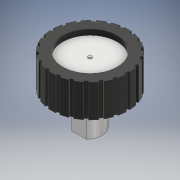
# Autodesk Inventor part: learnbotRueda
Saved by Autodesk Inventor 2017 (Build 210142000, 142)
## iProperties
Part Number: learnbotRueda
Material: Genérico
Document SubType Name: Modeling
Designer: rober
Density: 1 g/cm^3
Appearance: Valor por defecto
Author: rober
Autodesk Inventor part; units mm, degrees
ref_plane "YZ Plane" through (0, 0, 0) normal (1, 0, 0) x (0, 1, 0)
ref_plane "XZ Plane" through (0, 0, 0) normal (0, 1, 0) x (-1, 0, 0)
ref_plane "XY Plane" through (0, 0, 0) normal (0, 0, 1) x (1, 0, 0)
sketch "Boceto1" plane through (0, 0, 0) normal (0, 0, 1) x (1, 0, 0)
  circle A0 centre (0, 0.0001) radius 1.5
  line L0 (-0.1991, -2.0905) -> (0.1991, -2.0905)
  line L1 (0.3964, -2.0622) -> (0.7785, -1.9503)
  line L2 (0.9583, -1.8685) -> (1.2966, -1.6518)
  line L3 (0.7785, -1.9503) -> (0.7414, -1.8574)
  line L4 (0.9583, -1.8685) -> (0.9127, -1.7795)
  arc A1 (1.2349, -1.5731) -> (1.3772, -1.4502) centre (0, 0.0001) ccw
  arc A2 (-1.3773, -1.4502) -> (-1.235, -1.5731) centre (0, 0.0001) ccw
  arc A3 (-0.9128, -1.7795) -> (-0.7415, -1.8574) centre (0, 0.0001) ccw
  arc A4 (-0.3776, -1.964) -> (-0.1897, -1.9909) centre (0, 0.0001) ccw
  arc A5 (0.1896, -1.9909) -> (0.3775, -1.964) centre (0, 0.0001) ccw
  arc A6 (0.7414, -1.8574) -> (0.9127, -1.7795) centre (0, 0.0001) ccw
  line L5 (-1.2967, -1.6518) -> (-0.9584, -1.8685)
  line L6 (-0.7786, -1.9503) -> (-0.3964, -2.0622)
  line L7 (0.3775, -1.964) -> (0.3964, -2.0622)
  line L8 (0.1896, -1.9909) -> (0.1991, -2.0905)
  line L9 (-0.1897, -1.9909) -> (-0.1991, -2.0905)
  line L10 (-0.3776, -1.964) -> (-0.3964, -2.0622)
  line L11 (-1.235, -1.5731) -> (-1.2967, -1.6518)
  line L12 (-0.9584, -1.8685) -> (-0.9128, -1.7795)
  line L13 (-0.7415, -1.8574) -> (-0.7786, -1.9503)
  line L14 (1.2966, -1.6518) -> (1.2349, -1.5731)
  line L15 (-0.1991, 2.0906) -> (0.1991, 2.0906)
  line L16 (0.3964, 2.0623) -> (0.7785, 1.9504)
  line L17 (0.9583, 1.8686) -> (1.2966, 1.6519)
  line L18 (0.7785, 1.9504) -> (0.7414, 1.8575)
  line L19 (0.9583, 1.8686) -> (0.9127, 1.7796)
  arc A7 (1.3878, 1.4401) -> (1.2349, 1.5732) centre (-0.0001, 0) ccw
  arc A8 (-1.235, 1.5732) -> (-1.3879, 1.4401) centre (0, 0) ccw
  arc A9 (-0.7415, 1.8575) -> (-0.9128, 1.7796) centre (0, 0.0001) ccw
  arc A10 (-0.1897, 1.991) -> (-0.3776, 1.9641) centre (0, 0.0001) ccw
  arc A11 (0.3775, 1.9641) -> (0.1896, 1.991) centre (0, 0.0001) ccw
  arc A12 (0.9127, 1.7796) -> (0.7414, 1.8575) centre (0, 0.0001) ccw
  line L20 (-1.2967, 1.6519) -> (-0.9584, 1.8686)
  line L21 (-0.7786, 1.9504) -> (-0.3964, 2.0623)
  line L22 (0.3775, 1.9641) -> (0.3964, 2.0623)
  line L23 (0.1896, 1.991) -> (0.1991, 2.0906)
  line L24 (-0.1897, 1.991) -> (-0.1991, 2.0906)
  line L25 (-0.3776, 1.9641) -> (-0.3964, 2.0623)
  line L26 (-1.235, 1.5732) -> (-1.2967, 1.6519)
  line L27 (-0.9584, 1.8686) -> (-0.9128, 1.7796)
  line L28 (-0.7415, 1.8575) -> (-0.7786, 1.9504)
  line L29 (1.2966, 1.6519) -> (1.2349, 1.5732)
  line L30 (1.4461, -1.5227) -> (1.7075, -1.2223)
  line L31 (1.8148, -1.0565) -> (1.9828, -0.6915)
  line L32 (1.7075, -1.2223) -> (1.6262, -1.1641)
  line L33 (1.8148, -1.0565) -> (1.7284, -1.0062)
  arc A13 (1.6262, -1.1641) -> (1.7284, -1.0062) centre (0, 0.0001) ccw
  line L34 (1.3772, -1.4502) -> (1.4461, -1.5227)
  line L35 (2.039, -0.5021) -> (2.0973, -0.1046)
  line L36 (1.9828, -0.6915) -> (1.8884, -0.6585)
  line L37 (2.039, -0.5021) -> (1.9419, -0.4782)
  arc A14 (1.9975, -0.0996) -> (1.998, 0.0885) centre (0, 0.0001) ccw
  arc A15 (1.8884, -0.6585) -> (1.9419, -0.4782) centre (0, 0.0001) ccw
  line L38 (2.0973, -0.1046) -> (1.9975, -0.0996)
  line L39 (2.0979, 0.0929) -> (2.0427, 0.4873)
  line L40 (1.9878, 0.677) -> (1.8225, 1.0433)
  line L41 (2.0427, 0.4873) -> (1.9454, 0.4641)
  line L42 (1.9878, 0.677) -> (1.8932, 0.6448)
  arc A16 (1.9454, 0.4641) -> (1.8932, 0.6448) centre (0, 0.0001) ccw
  line L43 (1.998, 0.0885) -> (2.0979, 0.0929)
  arc A17 (1.7357, 0.9936) -> (1.6347, 1.1523) centre (0, 0.0001) ccw
  line L44 (1.8225, 1.0433) -> (1.7357, 0.9936)
  line L45 (1.7164, 1.2099) -> (1.4572, 1.5121)
  line L46 (1.4572, 1.5121) -> (1.3878, 1.4401)
  line L47 (1.6347, 1.1523) -> (1.7164, 1.2099)
  arc A18 (-1.3773, -1.4502) -> (-1.235, -1.5731) centre (0, 0.0001) ccw
  line L48 (-1.4462, -1.5227) -> (-1.7076, -1.2223)
  line L49 (-1.8149, -1.0565) -> (-1.9829, -0.6915)
  line L50 (-1.7076, -1.2223) -> (-1.6263, -1.1641)
  line L51 (-1.8149, -1.0565) -> (-1.7285, -1.0062)
  arc A19 (-1.7285, -1.0062) -> (-1.6263, -1.1641) centre (0, 0.0001) ccw
  line L52 (-1.3773, -1.4502) -> (-1.4462, -1.5227)
  line L53 (-2.0391, -0.5021) -> (-2.0974, -0.1046)
  line L54 (-1.9829, -0.6915) -> (-1.8885, -0.6585)
  line L55 (-2.0391, -0.5021) -> (-1.942, -0.4782)
  arc A20 (-1.9981, 0.0885) -> (-1.9976, -0.0996) centre (0, 0.0001) ccw
  arc A21 (-1.942, -0.4782) -> (-1.8885, -0.6585) centre (0, 0.0001) ccw
  line L56 (-2.0974, -0.1046) -> (-1.9976, -0.0996)
  line L57 (-2.098, 0.0929) -> (-2.0427, 0.4873)
  line L58 (-1.9879, 0.677) -> (-1.8226, 1.0433)
  line L59 (-2.0427, 0.4873) -> (-1.9455, 0.4641)
  line L60 (-1.9879, 0.677) -> (-1.8933, 0.6448)
  arc A22 (-1.8933, 0.6448) -> (-1.9455, 0.4641) centre (0, 0.0001) ccw
  line L61 (-1.9981, 0.0885) -> (-2.098, 0.0929)
  arc A23 (-1.6348, 1.1523) -> (-1.7358, 0.9936) centre (0, 0.0001) ccw
  line L62 (-1.8226, 1.0433) -> (-1.7358, 0.9936)
  line L63 (-1.7165, 1.2099) -> (-1.4573, 1.5121)
  line L64 (-1.4573, 1.5121) -> (-1.3879, 1.4401)
  line L65 (-1.6348, 1.1523) -> (-1.7165, 1.2099)
  circle A24 centre (0, 0.0001) radius 0.1
  point P0 (0, 0)
  constraints: 132 end point, 46 point on circle, 25 centre point
extrude "Extrusión1" add sketch "Boceto1" along normal blind 1.8 contours L9 A4 L10 L6 L13 A3 L12 L5 L11 A2 L52 L48 L50 A19 L51 L49 L54 A21 L55 L53 L56 A20 L61 L57 L59 A22 L60 L58 L62 A23 L65 L63 L64 A8 L26 L20 L27 A9 L28 L21 L25 A10 L24 L15 L23 A11 L22 L16 L18 A12 L19 L17 L29 A7 L46 L45 L47 A17 L44 L40 L42 A16 L41 L39 L43 A14 L38 L35 L37 A15 L36 L31 L33 A13 L32 L30 L34 A1 L14 L2 L4 A6 L3 L1 L7 A5 L8 L0
sketch "Boceto2" plane through (0, 0, 0) normal (0, 0, -1) x (-1, 0, 0)
  circle A0 centre (0, 0.0001) radius 1.5 projected
  point P0 (0, 0)
extrude "Extrusión2" add sketch "Boceto2" against normal blind 1.5
sketch "Boceto3" plane through (0, 0.0001, 1.5) normal (0, 0, 1) x (1, 0, 0)
  circle A0 centre (0, 0) radius 0.1
  point P0 (0, -0.0001)
  constraints: 1 centre point
extrude "Extrusión3" add sketch "Boceto3" along normal blind 0.05
sketch "Boceto4" plane through (0, 0, 0) normal (0, 0, -1) x (-1, 0, 0)
  line L0 (-0.4, 0.6001) -> (0.4, 0.6001)
  line L1 (0.4, -0.5999) -> (-0.4, -0.5999)
  arc A0 (-0.4, 0.6001) -> (-0.4, -0.5999) centre (0.195, 0.0001) ccw
  arc A1 (0.4, -0.5999) -> (0.4, 0.6001) centre (-0.195, 0.0001) ccw
  circle A2 centre (0, 0.0001) radius 0.1
  point P0 (0, 0)
  point P1 (-0.0001, 0)
  point P2 (0, 0)
  constraints: 4 end point, 4 point on circle, 3 centre point
extrude "Extrusión4" add sketch "Boceto4" along normal blind 1.9 contours L0 A1 L1 A0 | A2
sketch "Boceto5" plane through (0, 0, -1.9) normal (0, 0, -1) x (-1, 0, 0)
  line L0 (-0.4, 0.6001) -> (0.4, 0.6001)
  line L1 (0.4, -0.5999) -> (-0.4, -0.5999)
  arc A0 (-0.4, 0.6001) -> (-0.4, -0.5999) centre (0.195, 0.0001) ccw
  arc A1 (0.4, -0.5999) -> (0.4, 0.6001) centre (-0.195, 0.0001) ccw
  circle A2 centre (0, 0.0001) radius 0.1
  point P0 (0, 0)
  point P1 (-0.0001, 0)
  point P2 (0, 0)
  constraints: 4 end point, 4 point on circle, 3 centre point
extrude "Extrusión5" cut sketch "Boceto5" against normal blind 0.05 contours A2
sketch "Boceto6" plane through (0, 0, 0) normal (0, 0, -1) x (-1, 0, 0)
  circle A0 centre (0, 0.0001) radius 1.5 projected
  circle A1 centre (0, 0.0001) radius 0.1 projected
  line L0 (0.4, 0.6001) -> (-0.4, 0.6001) projected
  arc A2 (-0.4, 0.6001) -> (-0.4, -0.5999) centre (0.195, 0.0001) ccw projected
  line L1 (-0.4, -0.5999) -> (0.4, -0.5999) projected
  arc A3 (0.4, -0.5999) -> (0.4, 0.6001) centre (-0.195, 0.0001) ccw projected
  point P0 (0, 0)
extrude "Extrusión6" cut sketch "Boceto6" against normal blind 0.5 contours A0
